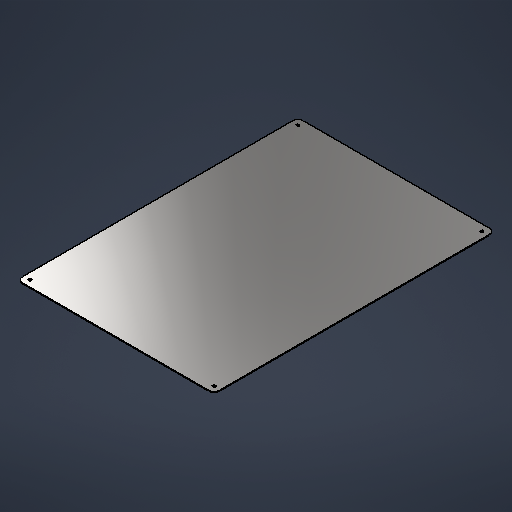
# Autodesk Inventor part: Side Panel
Saved by Autodesk Inventor 2026 (Build 300175050, 175E)
## iProperties
Created: 2025-05-19
Part Number: Side Panel
Material: Steel, Carbon
Document SubType Name: Sheet Metal
Designer: Joshua Eah
Density: 7.85 g/cm^3
Sheet Metal Rule: A36 Steel 20 ga
Appearance: Semi-Polished
Author: Joshua Eah
Autodesk Inventor part; units mm, degrees
ref_plane "YZ Plane" through (0, 0, 0) normal (1, 0, 0) x (0, 1, 0)
ref_plane "XZ Plane" through (0, 0, 0) normal (0, 1, 0) x (-1, 0, 0)
ref_plane "XY Plane" through (0, 0, 0) normal (0, 0, 1) x (1, 0, 0)
sketch "Sketch1" plane through (0, 0, 0) normal (0, 1, 0) x (-1, 0, 0)
  line L0 (0, 0) -> (-230, 0)
  line L1 (-230, 0) -> (-230, -328)
  line L2 (-230, -328) -> (0, -328)
  line L3 (0, -328) -> (0, 0)
  line L4 (-222.5, -7.5) -> (-7.5, -7.5) construction
  line L5 (-7.5, -7.5) -> (-7.5, -320.5) construction
  line L6 (-7.5, -320.5) -> (-222.5, -320.5) construction
  line L7 (-222.5, -320.5) -> (-222.5, -7.5) construction
  circle A0 centre (-7.5, -320.5) radius 1.6
  circle A1 centre (-222.5, -320.5) radius 1.6
  circle A2 centre (-222.5, -7.5) radius 1.6
  circle A3 centre (-7.5, -7.5) radius 1.6
  point P0 (-115, 0)
  dimension "d0" = 230
  dimension "d1" = 328
  dimension "d3" = 7.5
  dimension "d4" = 7.5
  dimension "d5" = 7.5
  dimension "d6" = 7.5
  dimension "d7" = 3.2
  constraints: 16 end point, 4 centre point, 4 coincident, 4 parallel, 3 equal radius, 2 horizontal, 2 perpendicular, 1 midpoint
  measures "d0" distance of L2.end L1.end
  measures "d1" distance of L1.end L0.end
  measures "d3" distance between parallel lines of L3 L5
  measures "d4" distance from line of point (-115, 0) L4
  measures "d5" distance between parallel lines of L1 L7
  measures "d6" distance between parallel lines of L2 L6
  measures "d7" diameter of A0
extrude "Plate1" add sketch "Sketch1" along normal blind 0.9119 contours L3 L2 L1 L0 | A0 | A1 | A2 | A3
hole "Hole1" at (222.5, 0, -320.5) at (7.5, 0, -320.5) at (7.5, 0, -7.5) at (222.5, 0, -7.5) direction (0, 1, 0) diameter 3.4036 end through all clearance for "Flat Head Machine Screw" size "M3" standard "Ansi Metric M Profile"
fillet "Corner Round1" radius 6.35 4 edges at (230, 0.4559, -328) (0, 0.4559, -328) (230, 0.4559, 0) (0, 0.4559, 0)
equation "\"d13\" = Thickness"
equation "\"d2\" = Thickness"
equation "\"BendRadius\" = Thickness"
equation "\"BendReliefWidth\" = Thickness"
equation "\"BendReliefDepth\" = 0.5 * Thickness"
equation "\"CornerReliefSize\" = 4 * Thickness"
equation "\"MinimumRemnant\" = 2 * Thickness"
equation "\"TransitionRadius\" = BendRadius"
equation "\"JacobiRadiusSize\" = BendRadius"
equation "\"GapSize\" = Thickness"
equation "\"Thickness\" = 0.91186"
body "Solid1"
